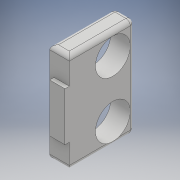
# Autodesk Inventor part: sonarMount
Saved by Autodesk Inventor 2017 (Build 210142000, 142)
## iProperties
Created: 2017-10-15
Part Number: sonarMount
Material: Generic
Document SubType Name: Modeling
Designer: Computus
Density: 1 g/cm^3
Appearance: Default
Author: Computus
## iProperties of the stored document sonarMount_3DPrint.ipt
Created: 2017-10-15
Part Number: sonarMount_3DPrint
Material: Generic
Document SubType Name: Modeling
Designer: Computus
Density: 1 g/cm^3
Appearance: Default
Author: Computus
Autodesk Inventor part; units mm, degrees
ref_plane "YZ Plane" through (0, 0, 0) normal (1, 0, 0) x (0, 1, 0)
ref_plane "XZ Plane" through (0, 0, 0) normal (0, 1, 0) x (-1, 0, 0)
ref_plane "XY Plane" through (0, 0, 0) normal (0, 0, 1) x (1, 0, 0)
sketch "Sketch1" plane through (0, 0, 0) normal (0, 1, 0) x (-1, 0, 0)
  line L0 (3, 12) -> (-4, 12)
  line L1 (-4, 12) -> (-4, -10.3)
  line L2 (-4, -10.3) -> (3, -10.3)
  line L3 (3, -10.3) -> (3, 12)
  point P0 (0, 0)
  dimension "d0" = 7
  dimension "d1" = 22.3
  constraints: 8 end point, 2 parallel, 1 horizontal, 1 perpendicular
  measures "d0" distance of L2.end L1.end
  measures "d1" distance of L1.end L0.end
extrude "Extrusion1" add sketch "Sketch1" along normal blind 2
sketch "Sketch2" plane through (0, 2, 0) normal (0, 1, 0) x (1, 0, 0)
  line L0 (-5, -24) -> (4, -24)
  line L1 (4, -24) -> (4, 21.5)
  line L2 (4, 21.5) -> (-5, 21.5)
  line L3 (-5, 21.5) -> (-5, -24)
  point P0 (0, 0)
  dimension "d4" = 45.5
  constraints: 8 end point, 2 parallel, 1 horizontal, 1 perpendicular
  measures "d4" distance of L1.end L0.end
extrude "Extrusion2" add sketch "Sketch2" along normal blind 30
sketch "Sketch3" plane through (4, 0, 12) normal (1, 0, 0) x (0, 0, -1)
  circle A0 centre (-2, 22) radius 8
  circle A1 centre (24, 22) radius 8
  point P0 (12, 0)
  dimension "d7" = 16
  dimension "d8" = 16
  dimension "d9" = 10
  constraints: 2 centre point
  measures "d7" diameter of A0
  measures "d8" diameter of A1
extrude "Extrusion3" cut sketch "Sketch3" against normal blind 30
fillet "Fillet1" radius 2 10 edges at (-0.5, 32, 24) (4, 32, 1.25) (-0.5, 32, -21.5) (-5, 32, 1.25) (-0.5, 2, 24) (4, 17, 24) (-5, 17, 24) (-0.5, 2, -21.5) (-5, 17, -21.5) (4, 17, -21.5)
body "Solid1"
